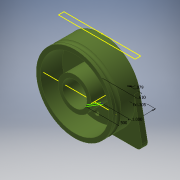
# Autodesk Inventor part: mounting plate
Saved by Autodesk Inventor 2018 (Build 220112000, 112)
## iProperties
Created: 2017-11-23
Part Number: mounting plate
Material: ABS Plastic
Document SubType Name: Modeling
Designer: prakh
Density: 1.06 g/cm^3
Appearance: Olive Green
Author: prakh
Autodesk Inventor part; units mm, degrees
ref_plane "YZ Plane" through (0, 0, 0) normal (1, 0, 0) x (0, 1, 0)
ref_plane "XZ Plane" through (0, 0, 0) normal (0, 1, 0) x (-1, 0, 0)
ref_plane "XY Plane" through (0, 0, 0) normal (0, 0, 1) x (1, 0, 0)
sketch "Sketch1" plane through (0, 0, 0) normal (0, 0, 1) x (1, 0, 0)
  circle A0 centre (0, 0) radius 44.45
  line L0 (-44.45, 44.45) -> (44.45, 44.45)
  line L1 (44.45, 44.45) -> (44.45, -44.45)
  line L2 (44.45, -44.45) -> (-44.45, -44.45)
  line L3 (-44.45, -44.45) -> (-44.45, 44.45)
  dimension "d0" = 88.9
  dimension "d1" = 88.9
  dimension "d2" = 88.9
  dimension "d3" = 44.45
  dimension "d4" = 44.45
  constraints: 8 end point, 2 parallel, 1 centre point, 1 coincident, 1 horizontal, 1 perpendicular
  measures "d0" diameter of A0
  measures "d1" distance of L1.end L2.end
  measures "d2" distance of L0.end L1.end
  measures "d3" distance from line of point (0, 0) L1
  measures "d4" distance from line of point (0, 0) L0
extrude "Extrusion1" add sketch "Sketch1" along normal blind 6.35
sketch "Sketch2" plane through (0, 0, 6.35) normal (0, 0, 1) x (1, 0, 0)
  circle A0 centre (0, 0) radius 46.0375
  circle A1 centre (0, 0) radius 44.45
  circle A2 centre (0, 0) radius 39.6875
  dimension "d8" = 1.5875
  dimension "d46" = 88.9
  dimension "d82" = 79.375
  constraints: 4 coincident, 3 centre point
  measures "d8" radial gap between concentric circles of A1 A0
  measures "d46" diameter of A1
  measures "d82" diameter of A2
extrude "Extrusion2" add sketch "Sketch2" along normal blind 25.4 contours A1
sketch "Sketch3" plane through (0, 0, 6.35) normal (0, 0, 1) x (1, 0, 0)
  circle A0 centre (0, 0) radius 14.2875
  dimension "d11" = 28.575
  constraints: 1 centre point, 1 coincident
  measures "d11" diameter of A0
extrude "Extrusion3" cut sketch "Sketch3" against normal blind 38.1
sketch "Sketch4" plane through (0, 0, 6.35) normal (0, 0, 1) x (1, 0, 0)
  circle A0 centre (0, 0) radius 14.2875 projected
  circle A1 centre (0, 0) radius 19.05
  dimension "d14" = 38.1
  constraints: 1 centre point, 1 coincident
  measures "d14" diameter of A1
extrude "Extrusion4" add sketch "Sketch4" along normal blind 25.4
sketch "Sketch7" plane through (0, 0, 6.35) normal (0, 0, 1) x (1, 0, 0)
  line L0 (44.45, 44.45) -> (0, 44.45) projected
  line L1 (-44.45, 44.45) -> (-44.45, 0) projected
  line L2 (-44.45, -44.45) -> (0, -44.45) projected
  line L3 (44.45, -44.45) -> (44.45, 0) projected
  line L4 (44.45, -44.45) -> (44.45, 44.45) projected
  line L5 (-44.45, 0) -> (-44.45, -44.45)
  line L6 (-44.45, -44.45) -> (0, -44.45)
  line L7 (44.45, -44.45) -> (-44.45, -44.45) projected
  line L8 (0, -44.45) -> (44.45, -44.45)
  line L9 (44.45, -44.45) -> (44.45, 0)
  arc A0 (-44.45, 0) -> (0, -44.45) centre (0, 0) ccw
  arc A1 (0, -44.45) -> (44.45, 0) centre (0, 0) ccw
  arc A2 (44.45, 0) -> (0, 44.45) centre (0, 0) ccw projected
  line L10 (44.45, 0) -> (44.45, 44.45) projected
  arc A3 (0, 44.45) -> (-44.45, 0) centre (0, 0) ccw projected
  line L11 (0, 44.45) -> (-44.45, 44.45) projected
  arc A4 (-44.45, 0) -> (0, -44.45) centre (0, 0) ccw projected
  line L12 (-44.45, 0) -> (-44.45, -44.45) projected
  arc A5 (0, -44.45) -> (44.45, 0) centre (0, 0) ccw projected
  line L13 (0, -44.45) -> (44.45, -44.45) projected
  point P0 (-44.4261, -1.4578)
  point P1 (44.4261, -1.4578)
  constraints: 8 end point, 4 point on circle, 2 centre point, 2 perpendicular, 1 horizontal, 1 vertical
extrude "Extrusion7" [suppressed]
sketch "Sketch8" plane through (0, 0, 0) normal (0, 1, 0) x (-1, 0, 0)
  line L0 (44.45, 6.35) -> (44.45, 31.75) projected
  arc A0 (44.45, 28.2575) -> (44.45, 22.5425) centre (45.974, 25.4) ccw
  line L1 (44.45, 31.75) -> (-44.45, 31.75) projected
  line L2 (0, -7.62) -> (0, 45.72) projected
  arc A1 (44.2147, 22.6811) -> (44.45, 28.2575) centre (45.974, 25.4) ccw
  point P0 (0, 0)
  dimension "d28" = 3.2385
  dimension "d31" = 19.05
  dimension "d45" = 1.7145
  constraints: 4 point on circle, 2 centre point, 2 point on line, 1 coincident
  measures "d28" radius of A0
  measures "d31" vertical distance of L0.start A0.centre
  measures "d45" distance edge to line of A0 L0
revolve "Revolution1" cut sketch "Sketch8" angle 360 about axis through (0, 0, -10) along (0, 0, 1) contours A0 L0
sketch "Sketch11" plane through (0, 0, 0) normal (0, 1, 0) x (-1, 0, 0)
  line L0 (-19.05, 6.35) -> (-19.05, 31.75) projected
  line L1 (-19.05, 38.1) -> (-26.605, 25.4)
  line L2 (-26.605, 25.4) -> (-23.8011, 25.4)
  line L3 (44.45, 28.2575) -> (-44.45, 28.2575) projected
  line L4 (-23.8011, 25.4) -> (-17.684, 35.6829)
  point P0 (0, 0)
  dimension "d43" = 25.4
  dimension "d44" = 12.7
  constraints: 6 end point, 2 parallel, 1 point on line
  measures "d43" distance from line of point (0, 0) L2
  measures "d44" vertical distance of L1.start L1.end
sketch "Sketch12" plane through (-44.45, 44.45, 0) normal (0, 1, 0) x (1, 0, 0)
  line L0 (0, 0) -> (88.9, 0) projected
  line L1 (0, 0) -> (0, -6.35) projected
  line L2 (44.45, -6.35) -> (0, -6.35) projected
  line L3 (88.9, 0) -> (88.9, -6.35) projected
  line L4 (88.9, -6.35) -> (44.45, -6.35) projected
  point P0 (44.45, 0)
sketch "Sketch13" plane through (0, 0, 0) normal (0, 0, -1) x (-1, 0, 0)
  circle A0 centre (0, 0) radius 44.45 projected
  arc A1 (-44.45, 0) -> (0, -44.45) centre (0, 0) ccw projected
  line L0 (-7.4513, 43.821) -> (0.0223, 44.45)
  line L1 (0.0223, 44.45) -> (0.2739, 41.4606)
  line L2 (0.2739, 41.4606) -> (-7.1997, 40.8316)
  line L3 (-7.1997, 40.8316) -> (-7.4513, 43.821)
  line L4 (4.1443, 44.2564) -> (11.526, 42.9296)
  line L5 (11.526, 42.9296) -> (10.9953, 39.9769)
  line L6 (10.9953, 39.9769) -> (3.6136, 41.3037)
  line L7 (3.6136, 41.3037) -> (4.1443, 44.2564)
  line L8 (0, 0) -> (0, 70.1731) construction
  line L9 (0, 0) -> (-12.1854, 69.107) construction
  line L10 (0, 0) -> (-24.0006, 65.9411) construction
  line L11 (0, 0) -> (-35.0865, 60.7717) construction
  line L12 (0, 0) -> (-45.1064, 53.7557) construction
  line L13 (0, 0) -> (-53.7557, 45.1064) construction
  line L14 (0, 0) -> (-60.7717, 35.0865) construction
  line L15 (0, 0) -> (-65.9411, 24.0006) construction
  line L16 (0, 0) -> (-69.107, 12.1854) construction
  line L17 (0, 0) -> (-70.1731, 0) construction
  line L18 (0, 0) -> (-69.107, -12.1854) construction
  line L19 (0, 0) -> (-65.9411, -24.0006) construction
  line L20 (0, 0) -> (-60.7717, -35.0865) construction
  line L21 (0, 0) -> (-53.7557, -45.1064) construction
  line L22 (0, 0) -> (-45.1064, -53.7557) construction
  line L23 (0, 0) -> (-35.0865, -60.7717) construction
  line L24 (0, 0) -> (-24.0006, -65.9411) construction
  line L25 (0, 0) -> (-12.1854, -69.107) construction
  line L26 (0, 0) -> (0, -70.1731) construction
  line L27 (0, 0) -> (12.1854, -69.107) construction
  line L28 (0, 0) -> (24.0006, -65.9411) construction
  line L29 (0, 0) -> (35.0865, -60.7717) construction
  line L30 (0, 0) -> (45.1064, -53.7557) construction
  line L31 (0, 0) -> (53.7557, -45.1064) construction
  line L32 (0, 0) -> (60.7717, -35.0865) construction
  line L33 (0, 0) -> (65.9411, -24.0006) construction
  line L34 (0, 0) -> (69.107, -12.1854) construction
  line L35 (0, 0) -> (70.1731, 0) construction
  line L36 (0, 0) -> (69.107, 12.1854) construction
  line L37 (0, 0) -> (65.9411, 24.0006) construction
  line L38 (0, 0) -> (60.7717, 35.0865) construction
  line L39 (0, 0) -> (53.7557, 45.1064) construction
  line L40 (0, 0) -> (45.1064, 53.7557) construction
  line L41 (0, 0) -> (35.0865, 60.7717) construction
  line L42 (0, 0) -> (24.0006, 65.9411) construction
  line L43 (0, 0) -> (12.1854, 69.107) construction
  arc A2 (0, 44.45) -> (-44.45, 0) centre (0, 0) ccw projected
  line L44 (44.45, 0) -> (43.7747, 7.7187)
  line L45 (43.7747, 7.7187) -> (40.7861, 7.4572)
  line L46 (40.7861, 7.4572) -> (41.4614, -0.2615)
  line L47 (41.4614, -0.2615) -> (44.45, 0)
  circle A3 centre (0, 0) radius 44.45 projected
  line L48 (44.2698, -3.9981) -> (41.3154, -3.4772)
  line L49 (41.3154, -3.4772) -> (40.013, -10.8632)
  line L50 (40.013, -10.8632) -> (42.9675, -11.3842)
  line L51 (44.2698, -3.9981) -> (42.9675, -11.3842)
  dimension "d53" = 7.5
  dimension "d54" = 3
  dimension "d55" = 3
  dimension "d56" = 7.5
  dimension "d59" = 360
  dimension "d61" = 15
  dimension "d95" = 3
  dimension "d98" = 15
  dimension "d99" = 7.5
  dimension "d100" = 3
  constraints: 104 end point, 7 parallel, 5 perpendicular, 5 point on circle, 2 point on line, 1 vertical, 117 other
  measures "d53" distance of L4.start L4.end
  measures "d54" distance of L4.end L5.end
  measures "d55" distance of L0.end L1.end
  measures "d56" distance of L0.start L0.end
  measures "d61" angle of L7 L1
  measures "d95" distance of L44.end L45.end
  measures "d98" angle of L48 L47
  measures "d99" distance of L48.start L50.end
  measures "d100" distance of L48.start L48.end
extrude "Extrusion11" cut sketch "Sketch13" against normal blind 13.35 contours L44 A0 | L47 L46 L45 L44 | L51 L50 L49 L48 | A0 L51
sketch "Sketch14" plane through (0, 0, 0) normal (0, 0, -1) x (-1, 0, 0)
  circle A0 centre (12.472, 29.1978) radius 2.7115
  circle A1 centre (-19.05, 25.4) radius 2.7115
  circle A2 centre (0.2661, -31.7489) radius 2.7115
  circle A3 centre (0, 0) radius 14.2875 projected
  dimension "d64" = 5.4229
  dimension "d71" = 31.75
  dimension "d72" = 31.75
  dimension "d73" = 31.75
  dimension "d74" = 31.75
  dimension "d75" = 60.325
  dimension "d76" = 25.4
  constraints: 3 centre point, 2 equal radius
  measures "d64" diameter of A1
  measures "d71" distance of A3.centre A2.centre
  measures "d72" distance of A1.centre point (0, 0)
  measures "d73" distance of A0.centre point (0, 0)
  measures "d74" distance of A0.centre A1.centre
  measures "d75" distance of A2.centre A1.centre
  measures "d76" vertical distance of A1.centre point (0, 0)
extrude "Extrusion12" cut sketch "Sketch14" against normal blind 25.4 contours A0 | A1 | A2
sketch "Sketch15" plane through (0, 0, 0) normal (0, 0, -1) x (-1, 0, 0)
  circle A0 centre (-31.75, 7.75) radius 1.004
  circle A1 centre (-31.75, -7.75) radius 1.004
  circle A2 centre (-31.75, 0) radius 6.35 projected
  point P0 (0, 0)
  dimension "d77" = 7.75
  dimension "d78" = 15.5
  dimension "d79" = 2.008
  constraints: 2 centre point, 2 vertical alignment, 1 equal radius
  measures "d77" distance of A2.centre A1.centre
  measures "d78" distance of A0.centre A1.centre
  measures "d79" diameter of A0
mirror "Mirror2" about plane through (0, 0, 0) normal (1, 0, 0) of "Extrusion12"
sketch "Sketch16" plane through (0, 0, 6.35) normal (0, 0, 1) x (1, 0, 0)
  circle A0 centre (28.575, 0) radius 5.95
  circle A1 centre (0, 0) radius 14.2875 projected
  dimension "d83" = 11.9
  dimension "d84" = 28.575
  constraints: 1 centre point, 1 horizontal alignment
  measures "d83" diameter of A0
  measures "d84" distance of A1.centre A0.centre
extrude "Extrusion14" cut sketch "Sketch16" against normal blind 25.4 contours A0
sketch "Sketch17" plane through (0, 0, 6.35) normal (0, 0, 1) x (1, 0, 0)
  line L0 (23.117, 5.6504) -> (23.117, 7.0495)
  line L1 (25.6612, 6.127) -> (25.6612, -0.8642)
  arc A0 (23.117, 7.0495) -> (25.6612, -0.8642) centre (0.8097, -4.4879) ccw
  arc A1 (25.6612, 6.127) -> (23.117, 5.6504) centre (24.359, 6.0493) ccw
  line L2 (26.9312, -0.7733) -> (26.9312, 5.9401)
  arc A2 (26.9312, 5.9401) -> (21.847, 5.4855) centre (24.359, 6.0493) ccw
  line L3 (21.847, 5.4855) -> (21.847, 11.4358)
  arc A3 (21.847, 11.4358) -> (26.9312, -0.7733) centre (0.8097, -4.4879) ccw
  point P0 (0, 0)
  dimension "d87" = 1.27
  constraints: 8 end point, 8 point on circle, 4 centre point, 2 vertical, 3 other
  measures "d87" radial gap between concentric circles of A0 A3
extrude "Extrusion15" [suppressed]
sketch "Sketch18" plane through (0, 0, 0) normal (0, 0, -1) x (-1, 0, 0)
  circle A0 centre (-28.575, 19) radius 1 projected
  circle A1 centre (-28.575, -8.3) radius 1 projected
  point P0 (0, 0)
extrude "Extrusion16" cut sketch "Sketch18" against normal blind 25.4
sketch "Sketch19" plane through (0, 0, 0) normal (0, 0, -1) x (-1, 0, 0)
  line L0 (-34.475, 16.6) -> (-22.675, 16.6) projected
  line L1 (-34.475, 16.6) -> (-34.475, -5.9) projected
  line L2 (-22.675, -5.9) -> (-22.675, 16.6) projected
  line L3 (-22.675, -5.9) -> (-34.475, -5.9) projected
  line L4 (-22.167, 17.108) -> (-34.983, 17.108)
  line L5 (-34.983, 17.108) -> (-34.983, -6.408)
  line L6 (-34.983, -6.408) -> (-22.167, -6.408)
  line L7 (-22.167, -6.408) -> (-22.167, 17.108)
  point P0 (0, 0)
  dimension "d92" = 0.508
  constraints: 8 end point, 3 other
  measures "d92" distance between parallel lines of L0 L4
extrude "Extrusion17" cut sketch "Sketch19" against normal blind 4.3 contours L0 L2 L3 L1 | L7 L6 L5 L4
sketch "Sketch20" plane through (0, 0, 0) normal (0, 0, -1) x (-1, 0, 0)
  line L0 (0, 44.45) -> (44.45, 44.45) projected
  line L1 (44.45, 44.45) -> (53.975, 44.45)
  line L2 (53.975, 44.45) -> (53.975, -44.45)
  line L3 (53.975, -44.45) -> (44.45, -44.45)
  line L4 (44.45, -44.45) -> (44.45, 44.45)
  line L5 (-44.45, 44.45) -> (-53.975, 44.45)
  line L6 (-53.975, 44.45) -> (-53.975, -44.45)
  line L7 (-53.975, -44.45) -> (-44.45, -44.45)
  line L8 (-44.45, -44.45) -> (-44.45, 44.45)
  line L9 (-44.45, -44.45) -> (44.45, -44.45) projected
  line L10 (-44.45, 44.45) -> (-44.45, -44.45) projected
  point P0 (0, 0)
  dimension "d101" = 9.525
  dimension "d102" = 9.525
  constraints: 16 end point, 4 parallel, 3 collinear, 2 horizontal, 2 perpendicular, 1 point on line
  measures "d101" distance of L6.end L7.end
  measures "d102" distance of L2.end L3.end
extrude "Extrusion18" add sketch "Sketch20" against normal up to surface (6.35 mm away)
sketch "Sketch21" plane through (0, 0, 6.35) normal (0, 0, 1) x (1, 0, 0)
  circle A0 centre (0, 0) radius 44.45 projected
  arc A1 (-43.7747, 7.7187) -> (-44.45, 0) centre (0, 0) ccw projected
  line L0 (0, -44.45) -> (53.975, -44.45) projected
  line L1 (53.975, -44.45) -> (43.6252, 8.5234)
  line L2 (-53.975, 44.45) -> (-53.975, -44.45) projected
  line L3 (-53.975, -44.45) -> (-43.6252, 8.5234)
  line L4 (53.975, 44.45) -> (53.975, -44.45) projected
  line L5 (53.975, -44.45) -> (53.975, 44.45)
  line L6 (53.975, 44.45) -> (0, 44.45)
  line L7 (-53.975, 44.45) -> (-53.975, -44.45)
  arc A2 (43.6252, 8.5234) -> (0, 44.45) centre (0, 0) ccw
  line L8 (0, 44.45) -> (-53.975, 44.45)
  arc A3 (0, 44.45) -> (-43.6252, 8.5234) centre (0, 0) ccw
  constraints: 12 end point, 6 point on circle, 2 centre point, 2 tangent, 1 coincident, 1 parallel
extrude "Extrusion19" cut sketch "Sketch21" against normal up to surface (6.35 mm away) contours A0 L6 L4 L1 | A0 L3 L2 L8
fillet "Fillet1" radius 6.35 2 edges at (53.975, -44.45, 3.175) (-53.975, -44.45, 3.175)
equation "\"d3\" = 0.5 * d1"
equation "\"d4\" = 0.5 * d2"
equation "\"d55\" = d54"
equation "\"d56\" = d53"
equation "\"d95\" = d54"
equation "\"d99\" = d53"
equation "\"d100\" = d54"
equation "\"d77\" = 0.5 * d78"
equation "\"d102\" = d101"
body "Solid1"
